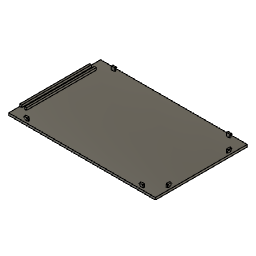
BOXlid (Autodesk Fusion 360 design; units mm, degrees)
Autodesk Fusion 360 part; units mm, degrees
sketch "Sketch1" plane through (0, 0, 0) normal (0, 0, 1) x (1, 0, 0)
  line L0 (0, 0) -> (134, 0)
  line L1 (134, 0) -> (134, 84)
  line L2 (134, 84) -> (0, 84)
  line L3 (0, 84) -> (0, 0)
  line L4 (2, 2) -> (132, 2)
  line L5 (132, 2) -> (132, 82)
  line L6 (132, 82) -> (2, 82)
  line L7 (0, 82) -> (1.8, 82)
  line L8 (1.8, 82) -> (1.8, 73.8)
  line L9 (1.8, 73.8) -> (0, 73.8)
  line L10 (0, 73.8) -> (0, 82)
  line L11 (0, 73.8) -> (1.8, 73.8)
  line L12 (1.8, 73.8) -> (1.8, 10.2)
  line L13 (1.8, 10.2) -> (0, 10.2)
  line L14 (0, 10.2) -> (0, 73.8)
  line L15 (4.4, 73.8) -> (4.4, 72.6661)
  line L16 (2, 72.6661) -> (2, 73.8)
  line L17 (4.4, 73.8) -> (6.2, 73.8)
  line L18 (6.2, 73.8) -> (6.2, 10.2)
  line L19 (6.2, 10.2) -> (4.4, 10.2)
  line L20 (4.4, 10.2) -> (4.4, 73.8)
  line L21 (2, 82) -> (1.8, 82)
  line L22 (1.8, 10.2) -> (1.8, 2)
  line L23 (2, 2) -> (1.8, 2)
  line L24 (1.8, 2) -> (12.8, 2)
  line L25 (12.8, 2) -> (15.8, 2)
  line L26 (15.8, 2) -> (15.8, 3)
  line L27 (15.8, 3) -> (12.8, 3)
  line L28 (12.8, 3) -> (12.8, 2)
  line L29 (12.8, 82) -> (15.8, 82)
  line L30 (15.8, 82) -> (15.8, 81)
  line L31 (15.8, 81) -> (12.8, 81)
  line L32 (12.8, 81) -> (12.8, 82)
  line L33 (132, 82) -> (121, 82)
  line L34 (132, 82) -> (132, 71)
  line L35 (121, 82) -> (118, 82)
  line L36 (118, 82) -> (118, 81)
  line L37 (118, 81) -> (121, 81)
  line L38 (121, 81) -> (121, 82)
  line L39 (132, 71) -> (131, 71)
  line L40 (131, 71) -> (131, 68)
  line L41 (131, 68) -> (132, 68)
  line L42 (132, 68) -> (132, 71)
  line L43 (132, 2) -> (132, 13)
  line L44 (132, 2) -> (121, 2)
  line L45 (132, 13) -> (131, 13)
  line L46 (131, 13) -> (131, 16)
  line L47 (131, 16) -> (132, 16)
  line L48 (132, 16) -> (132, 13)
  line L49 (121, 2) -> (118, 2)
  line L50 (118, 2) -> (118, 3)
  line L51 (118, 3) -> (121, 3)
  line L52 (121, 3) -> (121, 2)
  dimension "d1" = 134
  dimension "d2" = 84
  dimension "d33" = 130
  dimension "d34" = 80
  dimension "d35" = 1.8
  dimension "d36" = 8.2
  dimension "d37" = 63.6
  dimension "d38" = 2.4
  dimension "d39" = 1.8
  dimension "d41" = 11
  dimension "d42" = 3
  dimension "d43" = 1
  dimension "d44" = 1
  dimension "d45" = 11
  dimension "d46" = 11
  dimension "d47" = 3
  dimension "d48" = 11
  dimension "d49" = 11
  dimension "d50" = 1
  dimension "d51" = 3
  constraint horizontal L0
  constraint vertical L1
  constraint horizontal L2
  constraint vertical L3
  constraint coincident L0.start L3.end
  constraint horizontal L4
  constraint vertical L5
  constraint horizontal L6
  constraint horizontal L7
  constraint vertical L8
  constraint horizontal L9
  constraint vertical L10
  constraint coincident L3 L7.start
  constraint horizontal L11
  constraint vertical L12
  constraint horizontal L13
  constraint vertical L14
  constraint vertical L15
  constraint vertical L16
  constraint horizontal L17
  constraint vertical L18
  constraint horizontal L19
  constraint vertical L20
  constraint perpendicular L4 L22
  constraint perpendicular L22 L23
  constraint perpendicular L22 L24
  constraint horizontal L25
  constraint vertical L26
  constraint horizontal L27
  constraint vertical L28
  constraint horizontal L29
  constraint vertical L30
  constraint horizontal L31
  constraint vertical L32
  constraint coincident L6 L29.start
  constraint perpendicular L5 L33
  constraint perpendicular L6 L34
  constraint horizontal L35
  constraint vertical L36
  constraint horizontal L37
  constraint vertical L38
  constraint horizontal L39
  constraint vertical L40
  constraint horizontal L41
  constraint vertical L42
  constraint perpendicular L4 L43
  constraint perpendicular L5 L44
  constraint horizontal L45
  constraint vertical L46
  constraint horizontal L47
  constraint vertical L48
  constraint horizontal L49
  constraint vertical L50
  constraint horizontal L51
  constraint vertical L52
  measures "d1" distance of L0.start L0.end
  measures "d2" distance of L0.start L2.end
  measures "d33" distance of L4.start L4.end
  measures "d34" distance of L4.start L6.end
  measures "d35" distance of L7.start L7.end
  measures "d36" distance of L7.start L9.end
  measures "d37" distance of L9.end L13.end
  measures "d38" distance of L16.end L15.start
  measures "d39" distance of L15.start L17.end
  measures "d41" distance of L22.end L24.end
  measures "d42" distance of L24.end L25.end
  measures "d43" distance of L24.end L27.end
  measures "d44" distance of L29.start L31.end
  measures "d45" distance of L5.end L33.end
  measures "d46" distance of L5.end L34.end
  measures "d47" distance of L33.end L35.end
  measures "d48" distance of L4.end L43.end
  measures "d49" distance of L4.end L44.end
  measures "d50" distance of L43.end L45.end
  measures "d51" distance of L43.end L47.end
extrude "Extrude1" add sketch "Sketch1" along normal blind 2 contours L0 L1 L2 L3 L4 L5 L6 L7 L13 L21 L22 L23 L24 L25 L29 L33 L34 L35 L42 L43 L44 L48 L49 | L3 L9 L11 L12 L13 L14 | L3 L7 L8 L9 L10 L11 | L4 L5 L6 L8 L12 L21 L22 L23 L24 L26 L27 L28 L30 L31 L32 L33 L34 L36 L37 L38 L39 L40 L41 L43 L44 L45 L46 L47 L50 L51 L52 | L4 L25 L26 L27 L28 | L6 L29 L30 L31 L32 | L4 L49 L50 L51 L52 | L6 L35 L36 L37 L38 | L5 L45 L46 L47 L48 | L5 L39 L40 L41 L42 | L15 L17 L18 L19 L20
extrude "Extrude7" add sketch "Sketch1" along normal blind 5 contours L4 L25 L26 L27 L28 | L6 L29 L30 L31 L32 | L4 L49 L50 L51 L52 | L6 L35 L36 L37 L38 | L5 L45 L46 L47 L48 | L5 L39 L40 L41 L42
extrude "Extrude8" add sketch "Sketch1" along normal blind 4 contours L3 L9 L11 L12 L13 L14 | L15 L17 L18 L19 L20
sketch "Sketch8" plane through (0, 2, 0) normal (0, -1, 0) x (1, 0, 0)
  line L0 (12.8, 2) -> (15.8, 2)
  line L1 (15.8, 2) -> (15.8, 5)
  line L2 (15.8, 5) -> (12.8, 5)
  line L3 (12.8, 5) -> (12.8, 2)
  line L4 (12.8, 5) -> (15.8, 5)
  line L5 (15.8, 5) -> (15.8, 4)
  line L6 (15.8, 4) -> (12.8, 4)
  line L7 (12.8, 4) -> (12.8, 5)
  line L8 (118.0033, 5) -> (121.0033, 5)
  line L9 (121.0033, 5) -> (121.0033, 4)
  line L10 (121.0033, 4) -> (118.0033, 4)
  line L11 (118.0033, 4) -> (118.0033, 5)
  dimension "d56" = 1
  dimension "d57" = 3
  dimension "d58" = 1
  constraint horizontal L4
  constraint vertical L5
  constraint horizontal L6
  constraint vertical L7
  constraint coincident L2.end L3.start
  constraint horizontal L8
  constraint vertical L9
  constraint horizontal L10
  constraint vertical L11
  measures "d56" distance of L2.end L6.end
  measures "d57" distance of L8.start L8.end
  measures "d58" distance of L8.start L10.end
extrude "Extrude9" add sketch "Sketch8" along normal blind 1 contours L1 L2 L3 L4 L5 L6 L7 | L8 L9 L10 L11
sketch "Sketch9" plane through (132, 0, 0) normal (1, 0, 0) x (0, 1, 0)
  line L0 (13, 2) -> (16, 2)
  line L1 (16, 2) -> (16, 5)
  line L2 (16, 5) -> (13, 5)
  line L3 (13, 5) -> (13, 2)
  line L4 (13, 5) -> (16, 5)
  line L5 (16, 5) -> (16, 4)
  line L6 (16, 4) -> (13, 4)
  line L7 (13, 4) -> (13, 5)
  line L8 (68, 5) -> (71, 5)
  line L9 (71, 5) -> (71, 4)
  line L10 (71, 4) -> (68, 4)
  line L11 (68, 4) -> (68, 5)
  dimension "d61" = 3
  dimension "d62" = 1
  dimension "d63" = 3
  dimension "d64" = 1
  constraint horizontal L4
  constraint vertical L5
  constraint horizontal L6
  constraint vertical L7
  constraint coincident L2.end L3.start
  constraint horizontal L8
  constraint vertical L9
  constraint horizontal L10
  constraint vertical L11
  measures "d61" distance of L2.end L1.end
  measures "d62" distance of L2.end L6.end
  measures "d63" distance of L8.start L8.end
  measures "d64" distance of L8.start L10.end
extrude "Extrude10" add sketch "Sketch9" along normal blind 1 contours L1 L2 L3 L4 L5 L6 L7 | L8 L9 L10 L11
sketch "Sketch10" plane through (0, 82, 0) normal (0, 1, 0) x (-1, 0, 0)
  line L0 (-121, 2) -> (-118, 2)
  line L1 (-118, 2) -> (-118, 5)
  line L2 (-118, 5) -> (-121, 5)
  line L3 (-121, 5) -> (-121, 2)
  line L4 (-15.8, 5) -> (-12.8, 5)
  line L5 (-12.8, 5) -> (-12.8, 4)
  line L6 (-12.8, 4) -> (-15.8, 4)
  line L7 (-15.8, 4) -> (-15.8, 5)
  line L8 (-121, 5) -> (-118, 5)
  line L9 (-118, 5) -> (-118, 4)
  line L10 (-118, 4) -> (-121, 4)
  line L11 (-121, 4) -> (-121, 5)
  dimension "d67" = 3
  dimension "d68" = 1
  dimension "d69" = 3
  dimension "d70" = 1
  constraint horizontal L4
  constraint vertical L5
  constraint horizontal L6
  constraint vertical L7
  constraint horizontal L8
  constraint vertical L9
  constraint horizontal L10
  constraint vertical L11
  constraint coincident L2.end L3.start
  measures "d67" distance of L4.start L4.end
  measures "d68" distance of L4.start L6.end
  measures "d69" distance of L2.end L1.end
  measures "d70" distance of L2.end L10.end
extrude "Extrude11" add sketch "Sketch10" along normal blind 1 contours L1 L2 L3 L8 L9 L10 L11 | L4 L5 L6 L7
fillet "Fillet2" radius 0.5 12 edges at (119.5, 83, 5) (119.5, 83, 4) (133, 69.5, 5) (133, 69.5, 4) (133, 14.5, 5) (133, 14.5, 4) (119.5033, 1, 5) (14.3, 83, 5) (14.3, 83, 4) (14.3, 1, 5) (14.3, 1, 4) (119.5033, 1, 4)
equation "d35 = 2 mm - 0.2 mm"
equation "d37 = 80 mm - ( 8.2 * 2 ) * 1 mm"
equation "d41 = 15 mm - 3 mm - 1 mm"
equation "d52 = 3 mm + 2 mm"
equation "d54 = 2 mm + 2 mm"
